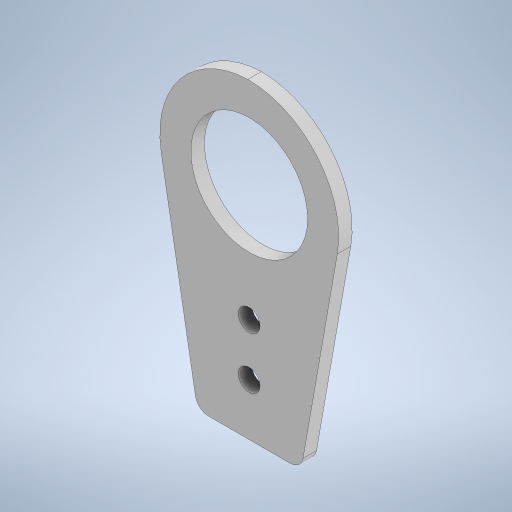
# Autodesk Inventor part: Arm Plate
Saved by Autodesk Inventor 2024 (Build 280153000, 153)
## iProperties
Created: 2023-10-19
Part Number: Arm Plate
Material: Generic
Document SubType Name: Modeling
Designer: ellen
Density: 1 g/cm^3
Appearance: Default
Author: ellen
Autodesk Inventor part; units mm, degrees
ref_plane "YZ Plane" through (0, 0, 0) normal (1, 0, 0) x (0, 1, 0)
ref_plane "XZ Plane" through (0, 0, 0) normal (0, 1, 0) x (-1, 0, 0)
ref_plane "XY Plane" through (0, 0, 0) normal (0, 0, 1) x (1, 0, 0)
sketch "Sketch1" plane through (0, 0, 0) normal (0, 0, 1) x (1, 0, 0)
  line L0 (44.45, 76.2) -> (0, 76.2)
  line L1 (0, 76.2) -> (0, 53.975)
  circle A0 centre (22.225, 53.975) radius 14.2875
  circle A1 centre (22.225, 25.4) radius 2.6543
  circle A2 centre (22.225, 12.7) radius 2.6543
  line L2 (0, 53.975) -> (9.525, 0)
  line L3 (44.45, 53.975) -> (34.925, 0)
  line L4 (9.525, 0) -> (34.925, 0)
  line L5 (44.45, 53.975) -> (44.45, 76.2)
  point P0 (0, 0)
  point P1 (22.225, 76.2)
  dimension "d0" = 44.45
  dimension "d2" = 28.575
  dimension "d3" = 5.3086
  dimension "d4" = 5.3086
  dimension "d5" = 22.225
  dimension "d6" = 50.8
  dimension "d7" = 63.5
  dimension "d8" = 22.225
  dimension "d9" = 22.225
  constraints: 12 end point, 3 centre point, 2 parallel, 1 horizontal, 1 midpoint, 1 perpendicular
  measures "d0" distance of L0.end L0.start
  measures "d2" diameter of A0
  measures "d3" diameter of A1
  measures "d4" diameter of A2
  measures "d5" distance of A0.centre point (22.225, 76.2)
  measures "d6" distance from line of L0 A1.centre
  measures "d7" distance from line of L0 A2.centre
  measures "d8" distance from line of L5 A1.centre
  measures "d9" distance from line of L5 A2.centre
extrude "Extrusion1" add sketch "Sketch1" along normal blind 3.302
fillet "Fillet9" radius 12.7 1 edges at (44.45, 53.975, 1.651)
fillet "Fillet10" radius 12.7 1 edges at (0, 53.975, 1.651)
fillet "Fillet11" radius 22.225 1 edges at (44.45, 76.2, 1.651)
fillet "Fillet12" radius 22.225 1 edges at (0, 76.2, 1.651)
fillet "Fillet13" radius 3.175 1 edges at (34.925, 0, 1.651)
fillet "Fillet14" radius 3.175 1 edges at (9.525, 0, 1.651)
body "Solid1"
